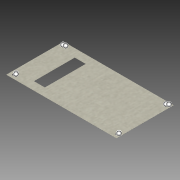
# Autodesk Inventor part: Paper Sheet
Saved by Autodesk Inventor 2015 (Build 190159000, 159)
## iProperties
Created: 2014-08-07
Part Number: Paper Sheet
Material: Paper
Document SubType Name: Modeling
Designer: simon
Density: 0.93 g/cm^3
Appearance: Cardboard - Chipboard
Author: simon
Autodesk Inventor part; units mm, degrees
ref_plane "YZ Plane" through (0, 0, 0) normal (1, 0, 0) x (0, 1, 0)
ref_plane "XZ Plane" through (0, 0, 0) normal (0, 1, 0) x (-1, 0, 0)
ref_plane "XY Plane" through (0, 0, 0) normal (0, 0, 1) x (1, 0, 0)
sketch "Sketch1" plane through (0, 0, 0) normal (0, 0, 1) x (1, 0, 0)
  line L0 (0, 0) -> (145.9, 0)
  line L1 (145.9, 0) -> (145.9, 75.9)
  line L2 (145.9, 75.9) -> (0, 75.9)
  line L3 (0, 75.9) -> (0, 0)
  dimension "d0" = 145.9
  dimension "d1" = 75.9
  constraints: 8 end point, 2 parallel, 1 horizontal, 1 perpendicular
  measures "d0" distance of L2.end L1.end
  measures "d1" distance of L1.end L0.end
extrude "Extrusion1" add sketch "Sketch1" along normal blind 0.1
sketch "Sketch2" plane through (0, 0, 0.1) normal (0, 0, 1) x (1, 0, 0)
  line L0 (0, 0) -> (145.9, 0) construction
  line L1 (145.9, 0) -> (145.9, 75.9) construction
  line L2 (145.9, 75.9) -> (0, 75.9) construction
  line L3 (0, 75.9) -> (0, 0) construction
  line L4 (141.05, 4.85) -> (4.85, 4.85) construction
  line L5 (4.85, 4.85) -> (4.85, 71.05) construction
  line L6 (4.85, 71.05) -> (141.05, 71.05) construction
  line L7 (141.05, 71.05) -> (141.05, 4.85) construction
  dimension "d4" = 4.85
  constraints: 8 end point, 4 coincident, 3 other
  measures "d4" distance between parallel lines of L0 L4
hole "Hole1" at (4.85, 71.05, 0.1) at (4.85, 4.85, 0.1) at (141.05, 4.85, 0.1) at (141.05, 71.05, 0.1) direction (0, 0, -1) diameter 3 end through all
sketch "Sketch3" plane through (0, 0, 0.1) normal (0, 0, 1) x (1, 0, 0)
  line L0 (25.8, 10.95) -> (40.2, 10.95)
  line L1 (40.2, 10.95) -> (40.2, 64.95)
  line L2 (40.2, 64.95) -> (25.8, 64.95)
  line L3 (25.8, 64.95) -> (25.8, 10.95)
  circle A0 centre (141.05, 4.85) radius 1.5 construction
  circle A1 centre (4.85, 71.05) radius 1.5 construction
  circle A2 centre (4.85, 4.85) radius 1.5 construction
  circle A3 centre (141.05, 71.05) radius 1.5 construction
  line L4 (0, 0) -> (145.9, 0) construction
  line L5 (145.9, 0) -> (145.9, 75.9) construction
  line L6 (145.9, 75.9) -> (0, 75.9) construction
  line L7 (0, 75.9) -> (0, 0) construction
  dimension "d20" = 105.7
  dimension "d21" = 14.4
  dimension "d22" = 54
  dimension "d23" = 10.95
  constraints: 8 end point, 2 parallel, 1 horizontal, 1 perpendicular
  measures "d20" distance between parallel lines of L5 L1
  measures "d21" distance between parallel lines of L1 L3
  measures "d22" distance between parallel lines of L0 L2
  measures "d23" distance between parallel lines of L6 L2
extrude "Extrusion2" cut sketch "Sketch3" against normal up to next
body "Solid1"
